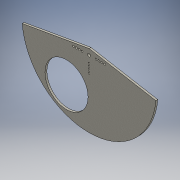
# Autodesk Inventor part: A0002
Saved by Autodesk Inventor 2017 (Build 210142000, 142)
## iProperties
Part Number: A0002
Material: 一般
Document SubType Name: Modeling
Designer: lygfy
Density: 1 g/cm^3
Appearance: 鋼 - 鑄造
Author: lygfy
Autodesk Inventor part; units mm, degrees
ref_plane "YZ Plane" through (0, 0, 0) normal (1, 0, 0) x (0, 1, 0)
ref_plane "XZ Plane" through (0, 0, 0) normal (0, 1, 0) x (-1, 0, 0)
ref_plane "XY Plane" through (0, 0, 0) normal (0, 0, 1) x (1, 0, 0)
sketch "草圖1" plane through (0, 0, 0) normal (0, 1, 0) x (-1, 0, 0)
  line L0 (0, 0) -> (5.9088, -1.0419) construction
  line L1 (0, 0) -> (-5.9088, -1.0419) construction
  arc A0 (5.9088, -1.0419) -> (-5.9088, -1.0419) centre (0, 0) ccw
  arc A1 (-68.9365, -12.1554) -> (68.9365, -12.1554) centre (0, 0) ccw
  line L2 (5.9088, -1.0419) -> (68.9365, -12.1554)
  line L3 (-5.9088, -1.0419) -> (-68.9365, -12.1554)
  circle A2 centre (23.5124, -38.3688) radius 22.5
  circle A3 centre (-23.5124, -38.3688) radius 22.5 construction
  arc A4 (-23.5124, -38.3688) -> (23.5124, -38.3688) centre (0, 0) ccw construction
  line L4 (23.5124, -38.3688) -> (0, 0) construction
  line L5 (-23.5124, -38.3688) -> (0, 0) construction
  line L6 (0, -85.2185) -> (0, 21.3111) construction
  line L7 (69.7247, -6.2018) -> (0, 6.0926)
  line L8 (0, 6.0926) -> (-69.7247, -6.2018)
  arc A5 (68.9365, -12.1554) -> (69.7247, -6.2018) centre (0, 0) ccw
  arc A6 (-69.7247, -6.2018) -> (-68.9365, -12.1554) centre (0, 0) ccw
  dimension "d0" = 12
  dimension "d1" = 45
  dimension "d3" = 45
  dimension "d5" = 160
  dimension "d6" = 63
  dimension "d7" = 70
  constraints: 16 end point, 10 point on circle, 7 centre point, 5 coincident, 2 collinear, 2 tangent, 1 concentric, 1 equal length, 1 parallel, 1 point on line, 4 other
  measures "d0" diameter of A0
  measures "d1" diameter of A2
  measures "d3" distance of L4.start L4.end
  measures "d5" angle of L3 L2
  measures "d6" angle of L5 L4
  measures "d7" distance of L0.start L2.end
extrude "擠出1" add sketch "草圖1" against normal blind 2
hole "孔1" at (0, 0, 0) direction (0, -1, 0) diameter 3.2 end through all
sketch "草圖2" plane through (0, 0, 0) normal (0, 1, 0) x (-1, 0, 0)
  arc A0 (-23.5124, -38.3688) -> (23.5124, -38.3688) centre (0, 0) ccw construction
  circle A1 centre (0, 0) radius 1.6 projected
  circle A2 centre (0, 0) radius 45
  constraints: 1 centre point, 1 coincident, 1 concentric
feature "擠出表面1" [suppressed]
sketch "草圖3" plane through (0, -2, 0) normal (0, -1, 0) x (1, 0, 0)
  circle A0 centre (0, -13.25) radius 0.75
  circle A1 centre (0, -16.25) radius 0.75
  circle A2 centre (0, -10.25) radius 0.75
  circle A3 centre (0, -7.25) radius 0.75
  line L0 (0, 0) -> (0, -16.25) construction
  circle A4 centre (0, 0) radius 1.6 construction
  circle A5 centre (13.25, 0) radius 0.75
  circle A6 centre (16.25, 0) radius 0.75
  circle A7 centre (10.25, 0) radius 0.75
  circle A8 centre (7.25, 0) radius 0.75
  circle A9 centre (0, 13.25) radius 0.75
  circle A10 centre (0, 16.25) radius 0.75
  circle A11 centre (0, 10.25) radius 0.75
  circle A12 centre (0, 7.25) radius 0.75
  circle A13 centre (-13.25, 0) radius 0.75
  circle A14 centre (-16.25, 0) radius 0.75
  circle A15 centre (-10.25, 0) radius 0.75
  circle A16 centre (-7.25, 0) radius 0.75
  dimension "d21" = 3
  dimension "d22" = 3
  dimension "d24" = 1.5
  dimension "d25" = 3
  dimension "d26" = 7.25
  dimension "d29" = 360
  constraints: 16 centre point, 3 equal radius, 3 point on line, 2 coincident, 2 end point, 1 vertical, 33 other
  measures "d21" distance of A2.centre A3.centre
  measures "d22" distance of A0.centre A2.centre
  measures "d24" diameter of A3
  measures "d25" distance of A0.centre L0.end
  measures "d26" distance of point (0, 0) A3.centre
hole "孔2" at (-7.25, -2, 0) at (-10.25, -2, 0) at (-13.25, -2, 0) at (-16.25, -2, 0) at (0, -2, -13.25) at (0, -2, -16.25) at (0, -2, -7.25) at (0, -2, -10.25) at (7.25, -2, 0) at (10.25, -2, 0) at (13.25, -2, 0) at (16.25, -2, 0) direction (0, 1, 0) diameter 2 end through all
